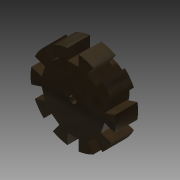
# Autodesk Inventor part: driveWheel01
Saved by Autodesk Inventor 2013 (Build 170138000, 138)
## iProperties
Created: 2013-01-21
Part Number: driveWheel01
Material: Wood (Maple)
Document SubType Name: Modeling
Designer: Nano
Density: 0.57 g/cm^3
Mass: 14.5813 g
Surface Area: 62.1495 cm^2
Volume: 25.5811 cm^3
Author: Nano
Autodesk Inventor part; units mm, degrees
ref_plane "YZ Plane" through (0, 0, 0) normal (1, 0, 0) x (0, 1, 0)
ref_plane "XZ Plane" through (0, 0, 0) normal (0, 1, 0) x (-1, 0, 0)
ref_plane "XY Plane" through (0, 0, 0) normal (0, 0, 1) x (1, 0, 0)
sketch "Sketch1" plane through (0, 0, 0) normal (0, 0, 1) x (1, 0, 0)
  circle A0 centre (0, 0) radius 1.95 projected
  circle A1 centre (0, 0) radius 23.9014
  point P0 (0, 0)
  dimension "d0" = 47.8028
  constraints: 1 centre point, 1 coincident
  measures "d0" diameter of A1
extrude "Extrusion1" add sketch "Sketch1" along normal blind 19.05
sketch "Sketch2" plane through (0, 0, 0) normal (0, 0, -1) x (-1, 0, 0)
  circle A0 centre (0, 0) radius 1.95 projected
  circle A1 centre (0, 0) radius 23.9014 projected
  circle A2 centre (0, 0) radius 12.7
  dimension "d3" = 25.4
  constraints: 1 centre point, 1 coincident
  measures "d3" diameter of A2
extrude "Extrusion2" cut sketch "Sketch2" against normal blind 6.35 contours A1
sketch "Sketch3" plane through (0, 0, 19.05) normal (0, 0, 1) x (1, 0, 0)
  circle A0 centre (0, 0) radius 23.9014 projected
  line L0 (-3.175, -17.5514) -> (3.175, -17.5514)
  line L1 (3.175, -17.5514) -> (3.175, -23.9014)
  line L2 (3.175, -23.9014) -> (-3.175, -23.9014)
  line L3 (-3.175, -23.9014) -> (-3.175, -17.5514)
  line L4 (0, 0) -> (0, -27.6264) construction
  point P0 (0, -17.5514)
  dimension "d6" = 6.35
  dimension "d7" = 6.35
  constraints: 10 end point, 3 parallel, 1 horizontal, 1 midpoint, 1 perpendicular, 1 point on line, 1 tangent
  measures "d6" distance of L1.end L2.end
  measures "d7" distance of L0.end L1.end
extrude "Extrusion3" cut sketch "Sketch3" against normal blind 12.7 contours L3 L0 L1 A0 | A0 L2 L3 | L1 L2 A0 picked at (0, -19.6681)
pattern_circular "Circular Pattern1" count 10 over 360 about axis through (0, 0, 0) along (0, 0, 1) of "Extrusion3"
body "Solid1"
